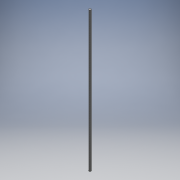
# Autodesk Inventor part: gevindstang
Saved by Autodesk Inventor 2018 (Build 220112000, 112)
## iProperties
Created: 2018-01-24
Part Number: gevindstang
Material: Steel
Document SubType Name: Modeling
Designer: MikkelS
Density: 7.85 g/cm^3
Appearance: Plate
Author: MikkelS
Autodesk Inventor part; units mm, degrees
ref_plane "YZ Plane" through (0, 0, 0) normal (1, 0, 0) x (0, 1, 0)
ref_plane "XZ Plane" through (0, 0, 0) normal (0, 1, 0) x (-1, 0, 0)
ref_plane "XY Plane" through (0, 0, 0) normal (0, 0, 1) x (1, 0, 0)
sketch "Sketch1" plane through (0, 0, 0) normal (0, 1, 0) x (-1, 0, 0)
  point P0 (0, 0)
sketch "Sketch2" plane through (0, 0, 0) normal (0, 0, 1) x (1, 0, 0)
  circle A0 centre (0, 0) radius 3
  dimension "d0" = 6
  constraints: 1 centre point, 1 coincident
  measures "d0" diameter of A0
extrude "Extrusion1" add sketch "Sketch2" along normal blind 393
thread "Thread1" size "M6x1" class "6g" standard "ANSI Metric M Profile" full length
body "Solid1"
